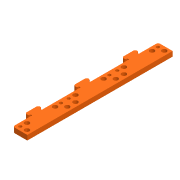
# Autodesk Inventor part: 40_Cube_XY_Table_Aliexpress_naked_puzzlebar
Saved by Autodesk Inventor 2022 (Build 260153000, 153)
## iProperties
Created: 2017-06-20
Part Number: 40_Cube_XY_Table_Aliexpress_naked_puzzlebar
Material: Generisch
Document SubType Name: Modeling
Designer: diederichbenedict
Density: 1 g/cm^3
Appearance: Glatt - Hellorange
Mass: 5.4697 g
Surface Area: 48.9743 cm^2
Volume: 5.4697 cm^3
Catalog Web Link: isInjectionmolded
Vendor: openUC2
d_part: 50,000 mm
d_o: 40,000 mm
d_i: 40,000 mm
Author: diederichbenedict
Autodesk Inventor part; units mm, degrees
ref_plane "YZ Plane" through (0, 0, 0) normal (1, 0, 0) x (0, 1, 0)
ref_plane "XZ Plane" through (0, 0, 0) normal (0, 1, 0) x (-1, 0, 0)
ref_plane "XY Plane" through (0, 0, 0) normal (0, 0, 1) x (1, 0, 0)
sketch "Skizze1" plane through (0, 0, 0) normal (0, 0, 1) x (1, 0, 0)
  line L0 (-17, 0) -> (-25, 0)
  line L1 (-25, 0) -> (-25, -23)
  line L2 (-23, -25) -> (0, -25)
  line L3 (0, -25) -> (0, -17)
  line L4 (-17, 0) -> (-17, -15)
  line L5 (-15, -17) -> (0, -17)
  arc A0 (-25, -23) -> (-23, -25) centre (-23, -23) ccw construction
  circle A1 centre (-20.8, -14.5) radius 2.4
  circle A2 centre (-14.5, -20.8) radius 2.4
  arc A3 (-17, -15) -> (-15, -17) centre (-15, -15) ccw
  circle A4 centre (-14.5, -20.8) radius 2.4 construction
  circle A5 centre (-20.8, -14.5) radius 2.4 construction
  line L6 (-30.4971, 0) -> (5.0828, 0) construction
  line L7 (0, -30.4971) -> (0, 5.0828) construction
  line L8 (-23, -25) -> (-25, -25)
  line L9 (-25, -23) -> (-25, -25)
  line L10 (0, -17) -> (0, 0)
  line L11 (0, 0) -> (-17, 0)
  point P0 (-17, -17)
  dimension "d278" = 25
  dimension "d279" = 25
  dimension "d2" = 8
  dimension "d281" = 8
  dimension "d282" = 2
  dimension "d286" = 4.8
  dimension "d_hole" = 4.8
  dimension "d290" = 20.8
  dimension "d" = 20.8
  dimension "d292" = 2
  dimension "d313" = 6.3
  dimension "d314" = 6.3
  dimension "d332" = 0
  constraints: 20 end point, 6 centre point, 6 point on line, 5 coincident, 4 point on circle, 4 tangent, 3 collinear, 2 horizontal, 2 parallel, 2 perpendicular
  measures "d278" distance of L2.end L8.end
  measures "d279" distance of L8.end L0.end
  measures "d2" distance between parallel lines of L4 L1
  measures "d281" distance between parallel lines of L2 L5
  measures "d282" radius of A0
  measures "d286" diameter of A1
  measures "d_hole" diameter of A2
  measures "d290" distance from line of L0 A2.centre
  measures "d" distance from line of L3 A1.centre
  measures "d292" radius of A3
  measures "d313" horizontal distance of A1.centre A2.centre
  measures "d314" horizontal distance of A1.centre A2.centre
  measures "d332" radial gap between concentric circles of A1 A5
extrude "Extrusion1" add sketch "Skizze1" along normal blind 5
mirror "Mirror6" about plane through (0, 0, 0) normal (0, 1, 0) of "Extrusion1"
sketch "Sketch26" plane through (0, 0, 5) normal (0, 0, 1) x (1, 0, 0)
  line L0 (-25, 25) -> (0, 25) projected
  line L1 (-25, -25) -> (-25, 25) projected
  line L2 (-25, -25) -> (0, -25) projected
  line L3 (-25, -23) -> (-25, 23) projected
  line L4 (-28.6, -7) -> (-28.6, -7)
  line L5 (-30.6, -5) -> (-30.6, 5)
  line L6 (-28.6, 7) -> (-28.6, 7)
  line L7 (-25, 16.8311) -> (-25, -7)
  line L8 (-26.3639, 5) -> (-25, 5)
  line L9 (-25, -5) -> (-26.3639, -5)
  arc A0 (-30.6, -5) -> (-28.6, -7) centre (-28.6, -5) ccw
  arc A1 (-28.6, -7) -> (-26.6124, -5.2222) centre (-28.6, -5) ccw
  arc A2 (-28.6, 7) -> (-30.6, 5) centre (-28.6, 5) ccw
  arc A3 (-26.6124, 5.2222) -> (-28.6, 7) centre (-28.6, 5) ccw
  arc A4 (-26.3639, -5) -> (-26.6124, -5.2222) centre (-26.3639, -5.25) ccw
  arc A5 (-26.6124, 5.2222) -> (-26.3639, 5) centre (-26.3639, 5.25) ccw
  line L10 (-37.2171, 0) -> (6.2028, 0) projected
  line L11 (0, -25) -> (0, 25) projected
  point P0 (0, 0)
  point P1 (-24.0313, 1.861)
  point P2 (-28.6, -7)
  point P3 (-25, -5)
  point P4 (-25, 5)
  point P5 (-28.6, 7)
  dimension "d293" = 5.6
  dimension "d300" = 2
  dimension "d301" = 0.25
  dimension "d365" = 7
  dimension "d367" = 7
  dimension "d385" = 5
  dimension "d386" = 5
  constraints: 12 end point, 12 point on circle, 10 tangent, 6 centre point, 4 equal radius, 3 parallel, 2 coincident, 2 point on line, 1 horizontal, 1 perpendicular, 1 other
  measures "d293" distance between parallel lines of L1 L5
  measures "d300" radius of A0
  measures "d301" radius of A4
  measures "d385" distance of the line from the sketch origin of L9
  measures "d386" distance of the line from the sketch origin of L8
extrude "Extrusion13" add sketch "Sketch26" against normal up to surface (5 mm away) contours L10 L5 A2 A3 A5 L8 L1 | L1 L9 A4 A1 A0 L5 L10
sketch "Skizze36" plane through (0, 0, 5) normal (0, 0, 1) x (1, 0, 0)
  line L0 (30.9789, 27.5712) -> (-10, 27.5712)
  line L1 (-10, 27.5712) -> (-10, -32.2955)
  line L2 (-10, -32.2955) -> (30.9789, -32.2955)
  line L3 (30.9789, -32.2955) -> (30.9789, 27.5712)
  line L4 (-25, 23) -> (-25, 5) projected
  point P0 (0, 0)
  dimension "d401" = 15
  constraints: 8 end point, 2 parallel, 1 horizontal, 1 perpendicular
  measures "d401" distance between parallel lines of L1 L4
extrude "Extrusion19" cut sketch "Skizze36" against normal blind 10
pattern_linear "Rechteckige Anordnung8" count 3 spacing 50 along (0, 1, 0) of "Extrusion1", "Mirror6", "Extrusion13", "Extrusion19"
fillet "Rundung6" radius 2 2 edges at (-25, -25, 2.5) (-25, 125, 2.5)
sketch "Skizze37" plane through (0, 0, 0) normal (0, 0, -1) x (-1, 0, 0)
  arc A0 (23.1, -20.49) -> (20.5755, -23.0145) centre (21.2, -21.1145) ccw projected
  arc A1 (20.7515, 22.8345) -> (23.1, 20.261) centre (21.2, 20.8855) ccw projected
  arc A2 (23.1, 29.51) -> (20.5755, 26.9855) centre (21.2, 28.8855) ccw projected
  arc A3 (20.7515, 72.8345) -> (23.1, 70.261) centre (21.2, 70.8855) ccw projected
  arc A4 (23.1, 79.51) -> (20.5755, 76.9855) centre (21.2, 78.8855) ccw projected
  arc A5 (20.7515, 122.8345) -> (23.1, 120.261) centre (21.2, 120.8855) ccw projected
  point P0 (0, 0)
hole "Bohrung8" at (-21.2, 120.8855, 0) at (-21.2, 78.8855, 0) at (-21.2, 70.8855, 0) at (-21.2, 28.8855, 0) at (-21.2, 20.8855, 0) at (-21.2, -21.1145, 0) direction (0, 0, 1) diameter 3.2 end through all
equation "\"d_i\" = 40"
equation "\"d_o\" = 40"
equation "\"d_part\" = 50"
equation "\"d6\" = 0"
equation "\"d7\" = 0"
equation "\"d8\" = 0"
equation "\"d9\" = 0"
equation "\"d13\" = 0"
equation "\"d14\" = 0"
equation "\"d20\" = 0"
equation "\"d21\" = 0"
equation "\"d22\" = 0"
equation "\"d23\" = 0"
equation "\"d24\" = 0"
equation "\"d25\" = 3"
equation "\"d26\" = 0"
equation "\"d27\" = 0"
equation "\"d28\" = 0"
equation "\"d29\" = 0"
equation "\"d30\" = 0"
equation "\"d31\" = 0"
equation "\"d32\" = 0"
equation "\"d33\" = 0"
equation "\"d34\" = 0"
equation "\"d46\" = 0"
equation "\"d47\" = 0"
equation "\"d48\" = 0"
equation "\"d50\" = 0"
equation "\"d51\" = 0"
equation "\"d52\" = 0"
equation "\"d53\" = 0"
equation "\"d54\" = 0"
equation "\"d55\" = 0"
equation "\"d56\" = 0"
equation "\"d57\" = 0"
equation "\"d58\" = 0"
equation "\"d59\" = 0"
equation "\"magnet_offset\" = 0"
equation "\"screw_offset\" = 0"
equation "\"mal_puzzle_offset\" = 0"
equation "\"fem_puzzle_offset\" = 0"
